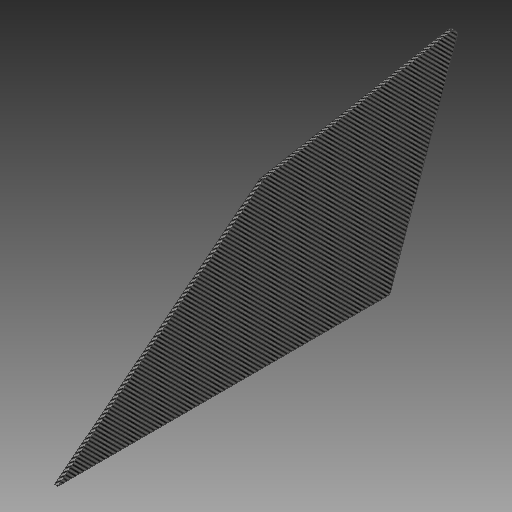
# Autodesk Inventor part: stay_middle
Saved by Autodesk Inventor 2018.1 (Build 221171000, 171)
## iProperties
Created: 2017-10-18
Part Number: stay_middle
Material: CFRP
Document SubType Name: Modeling
Designer: kuwano
Density: 1.43 g/cm^3
Appearance: カーボンファイバー
Mass: 158.571 g
Surface Area: 766.32 cm^2
Volume: 110.889 cm^3
Author: kuwano
Autodesk Inventor part; units mm, degrees
ref_plane "YZ Plane" through (0, 0, 0) normal (1, 0, 0) x (0, 1, 0)
ref_plane "XZ Plane" through (0, 0, 0) normal (0, 1, 0) x (-1, 0, 0)
ref_plane "XY Plane" through (0, 0, 0) normal (0, 0, 1) x (1, 0, 0)
sketch "スケッチ1" plane through (0, 0, 0) normal (1, 0, 0) x (0, 1, 0)
  line L0 (-90, 263.8963) -> (-90, -36.1037)
  line L1 (-90, -36.1037) -> (90, -100)
  line L2 (-126, 0) -> (126, 0) projected
  line L3 (0, -172.7793) -> (0, 336.6756) projected
  line L4 (-90, 263.8963) -> (56.4999, 78.6159)
  line L5 (56.4999, 78.6159) -> (90, -100)
  dimension "d0" = 300
  dimension "d5" = 90
  dimension "d6" = 100
  dimension "d7" = 90
  constraints: 9 end point, 1 vertical
  measures "d0" distance of L0.end L0.start
  measures "d5" distance between parallel lines of L0 L3
  measures "d6" distance from line of L2 L1.end
  measures "d7" distance from line of L3 L1.end
extrude "押し出し1" add sketch "スケッチ1" along normal blind 3
fillet "フィレット1" radius 5 1 edges at (1.5, 90, -100)
